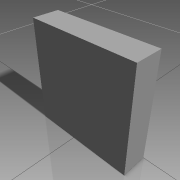
# Autodesk Inventor part: Cooler
Saved by Autodesk Inventor 2013 (Build 170138000, 138)
## iProperties
Created: 2014-04-26
Part Number: Cooler
Material: Generic
Document SubType Name: Modeling
Designer: spichelh
Density: 1 g/cm^3
Author: spichelh
Autodesk Inventor part; units mm, degrees
ref_plane "YZ Plane" through (0, 0, 0) normal (1, 0, 0) x (0, 1, 0)
ref_plane "XZ Plane" through (0, 0, 0) normal (0, 1, 0) x (-1, 0, 0)
ref_plane "XY Plane" through (0, 0, 0) normal (0, 0, 1) x (1, 0, 0)
sketch "Sketch1" plane through (0, 0, 0) normal (0, 0, 1) x (1, 0, 0)
  line L0 (-16.7714, -46.9047) -> (23.2286, -46.9047)
  line L1 (23.2286, -46.9047) -> (23.2286, -6.9047)
  line L2 (23.2286, -6.9047) -> (-16.7714, -6.9047)
  line L3 (-16.7714, -6.9047) -> (-16.7714, -46.9047)
  line L4 (-16.7714, -46.9047) -> (23.2286, -6.9047) construction
  line L5 (23.2286, -46.9047) -> (-16.7714, -6.9047) construction
  point P0 (0, 0)
  point P1 (3.2286, -26.9047)
  dimension "d0" = 40
  dimension "d1" = 40
  constraints: 12 end point, 2 midpoint, 2 parallel, 1 horizontal, 1 perpendicular
  measures "d0" distance of L2.end L1.end
  measures "d1" distance of L1.end L0.end
extrude "Extrusion1" add sketch "Sketch1" along normal blind 10
body "Solid1"
